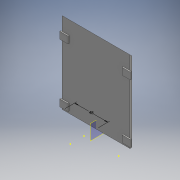
# Autodesk Inventor part: CAP1
Saved by Autodesk Inventor 2016 (Build 200138000, 138)
## iProperties
Created: 2017-07-01
Part Number: CAP1
Material: Generic
Document SubType Name: Modeling
Designer: ALIREZA
Density: 1 g/cm^3
Appearance: Default
Author: ALIREZA
Autodesk Inventor part; units mm, degrees
ref_plane "YZ Plane" through (0, 0, 0) normal (1, 0, 0) x (0, 1, 0)
ref_plane "XZ Plane" through (0, 0, 0) normal (0, 1, 0) x (-1, 0, 0)
ref_plane "XY Plane" through (0, 0, 0) normal (0, 0, 1) x (1, 0, 0)
sketch "Sketch1" plane through (0, 0, 0) normal (0, 0, 1) x (1, 0, 0)
  line L0 (-52.5, -20) -> (52.5, -20)
  line L1 (52.5, 20) -> (-52.5, 20)
  line L2 (-52.5, -20) -> (52.5, 20) construction
  line L3 (52.5, -20) -> (-52.5, 20) construction
  line L4 (-50, 17.5) -> (50, 17.5)
  line L5 (50, -17.5) -> (-50, -17.5)
  line L6 (-50, 17.5) -> (50, -17.5) construction
  line L7 (50, 17.5) -> (-50, -17.5) construction
  line L8 (60.5, 0) -> (60.5, 8)
  line L9 (60.5, 8) -> (52.5, 20)
  line L10 (60.5, 0) -> (60.5, -8)
  line L11 (60.5, -8) -> (52.5, -20)
  line L12 (50, -17.5) -> (56.5426, -7.6861)
  line L13 (56.5426, -7.6861) -> (56.5426, 7.6861)
  line L14 (56.5426, 7.6861) -> (50, 17.5)
  line L15 (0, 0) -> (0, 38.4543) construction
  line L16 (-60.5, 0) -> (-60.5, 8)
  line L17 (-60.5, 8) -> (-52.5, 20)
  line L18 (-60.5, 0) -> (-60.5, -8)
  line L19 (-60.5, -8) -> (-52.5, -20)
  line L20 (-50, -17.5) -> (-56.5426, -7.6861)
  line L21 (-56.5426, -7.6861) -> (-56.5426, 7.6861)
  line L22 (-56.5426, 7.6861) -> (-50, 17.5)
  dimension "d0" = 105
  dimension "d1" = 40
  dimension "d2" = 100
  dimension "d3" = 35
  dimension "d5" = 8
  dimension "d6" = 8
  constraints: 46 end point, 5 parallel, 5 symmetric about line, 4 midpoint, 2 horizontal, 2 point on line, 1 vertical
  measures "d0" distance of L1.end L1.start
  measures "d1" distance of L1.start L0.end
  measures "d2" distance of L5.start L5.end
  measures "d3" distance of L4.end L5.start
  measures "d5" distance of L8.start L8.end
  measures "d6" distance of L8.start L10.end
extrude "Extrusion1" add sketch "Sketch1" along normal blind 120
sketch "Sketch2" plane through (0, 0, 120) normal (0, 0, 1) x (1, 0, 0)
  line L0 (-56.5426, 7.6861) -> (-50, 17.5) projected
  line L1 (-50, 17.5) -> (50, 17.5) projected
  line L2 (50, 17.5) -> (56.5426, 7.6861) projected
  line L3 (56.5426, 7.6861) -> (56.5426, -7.6861) projected
  line L4 (56.5426, -7.6861) -> (50, -17.5) projected
  line L5 (50, -17.5) -> (-50, -17.5) projected
  line L6 (-50, -17.5) -> (-56.5426, -7.6861) projected
  line L7 (-56.5426, -7.6861) -> (-56.5426, 7.6861) projected
  point P0 (0, 0)
extrude "Extrusion2" add sketch "Sketch2" against normal blind 2.5
sketch "Sketch3" plane through (0, 0, 0) normal (0, 0, -1) x (-1, 0, 0)
  point P0 (0, 0)
fillet "Fillet1" radius 1 2 edges at (0, -17.5, 117.5) (0, 17.5, 117.5)
chamfer "Chamfer1" distance 5 angle 45 6 edges at (0, 20, 120) (-56.5, 14, 120) (-56.5, -14, 120) (0, -20, 120) (56.5, 14, 120) (56.5, -14, 120)
sketch "Sketch4" plane through (-52.5, -20, 0) normal (0, -1, 0) x (1, 0, 0)
  point P0 (52.5, 0)
sketch "Sketch5" plane through (0, 0, 0) normal (0, 0, -1) x (-1, 0, 0)
  line L0 (-50, 17.5) -> (50, 17.5) projected
  line L1 (-50, 17.5) -> (-50, 24.1033)
  line L2 (-50, 24.1033) -> (-71.4575, 13.1576)
  line L3 (-71.4575, 13.1576) -> (-66.6293, -23.8647)
  line L4 (-66.6293, -23.8647) -> (1.9313, -29.9815)
  line L5 (1.9313, -29.9815) -> (78.5389, -23.8647)
  line L6 (78.5389, -23.8647) -> (75.9786, 8.2013)
  line L7 (75.9786, 8.2013) -> (50, 28.9973)
  line L8 (50, 28.9973) -> (50, 17.5)
  point P0 (0, 0)
  constraints: 16 end point, 1 parallel, 1 perpendicular, 1 vertical
extrude "Extrusion3" cut sketch "Sketch5" against normal blind 120
sketch "Sketch6" plane through (50, 17.5, 0) normal (1, 0, 0) x (0, 0, -1)
  point P0 (0, -17.5)
sketch "Sketch7" plane through (0, 0, 0) normal (0, 0, -1) x (-1, 0, 0)
  line L0 (-50, 20) -> (50, 20) construction
  line L1 (0, 20) -> (48, 20) construction
  point P0 (0, 0)
  dimension "d17" = 48
  constraints: 2 end point, 1 midpoint, 1 point on line
  measures "d17" distance of L1.start L1.end
sketch "Sketch8" plane through (0, 0, 0) normal (0, 0, -1) x (-1, 0, 0)
  line L0 (49, 24.3422) -> (51, 24.3422)
  line L1 (51, 24.3422) -> (51, 15.6578)
  line L2 (51, 15.6578) -> (49, 15.6578)
  line L3 (49, 15.6578) -> (49, 24.3422)
  line L4 (-50, 20) -> (50, 20) projected
  line L5 (49, 24.3422) -> (51, 15.6578) construction
  line L6 (51, 24.3422) -> (49, 15.6578) construction
  point P0 (0, 0)
  dimension "d18" = 2
  constraints: 12 end point, 2 midpoint, 2 parallel, 1 horizontal, 1 perpendicular
  measures "d18" distance of L1.end L2.end
extrude "Extrusion4" cut sketch "Sketch8" against normal blind 120
ref_plane "Work Plane1" through (0, 20, 0) normal (-1, 0, 0) x (0, -1, 0)
mirror "Mirror1" about plane through (0, 20, 0) normal (-1, 0, 0) of "Extrusion4"
sketch "Sketch9" plane through (49, 17.5, 0) normal (1, 0, 0) x (0, 0, -1)
  line L0 (-2.9947, 0) -> (-12.9947, 0)
  line L1 (-12.9947, 0) -> (-12.9947, -1.5)
  line L2 (-12.9947, -1.5) -> (-2.9947, -1.5)
  line L3 (-2.9947, -1.5) -> (-2.9947, 0)
  line L4 (-115, 2.5) -> (-100, 2.5)
  line L5 (-97.7055, -1.5) -> (-87.7055, -1.5)
  line L6 (-87.7055, -1.5) -> (-87.7055, 0)
  line L7 (-87.7055, 0) -> (-97.7055, 0)
  line L8 (-97.7055, 0) -> (-97.7055, -1.5)
  point P0 (0, -17.5)
  point P1 (0, 2.5)
  dimension "d21" = 10
  dimension "d22" = 1.5
  dimension "d23" = 15
  dimension "d24" = 10
  constraints: 18 end point, 4 parallel, 2 horizontal, 2 perpendicular
  measures "d21" distance of L2.end L1.end
  measures "d22" distance of L1.end L0.end
  measures "d23" distance of L4.start L4.end
  measures "d24" distance of L7.end L6.end
extrude "Extrusion5" add sketch "Sketch9" along normal blind 2 and the other way blind 10
mirror "Mirror2" about plane through (0, 20, 0) normal (-1, 0, 0) of "Extrusion5"
body "Solid1"
